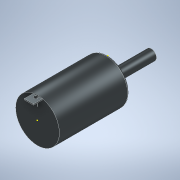
# Autodesk Inventor part: DC MOTOR
Saved by Autodesk Inventor 2022 (Build 260153000, 153)
## iProperties
Created: 2022-08-22
Part Number: DC MOTOR
Material: Iron, Gray
Document SubType Name: Modeling
Designer: Sachin
Density: 7.15 g/cm^3
Appearance: Iron Gray
Author: Sachin
Autodesk Inventor part; units mm, degrees
ref_plane "YZ Plane" through (0, 0, 0) normal (1, 0, 0) x (0, 1, 0)
ref_plane "XZ Plane" through (0, 0, 0) normal (0, 1, 0) x (-1, 0, 0)
ref_plane "XY Plane" through (0, 0, 0) normal (0, 0, 1) x (1, 0, 0)
sketch "Sketch1" plane through (0, 0, 0) normal (0, 0, 1) x (1, 0, 0)
  circle A0 centre (0, 0) radius 12.5
  dimension "d0" = 25
  constraints: 1 centre point, 1 coincident
  measures "d0" diameter of A0
extrude "Extrusion1" add sketch "Sketch1" along normal blind 40
sketch "Sketch2" plane through (0, 0, 40) normal (0, 0, 1) x (1, 0, 0)
  point P0 (0, 0)
sketch "Sketch3" plane through (0, 0, 40) normal (0, 0, 1) x (1, 0, 0)
  line L0 (-2.5708, 11.9347) -> (2.7411, 11.9347)
  line L1 (2.7411, 11.9347) -> (2.7411, 11.3559)
  line L2 (2.7411, 11.3559) -> (-2.5708, 11.3559)
  line L3 (-2.5708, 11.3559) -> (-2.5708, 11.9347)
  point P0 (0, 0)
  constraints: 8 end point, 2 parallel, 1 horizontal, 1 perpendicular
extrude "Extrusion2" add sketch "Sketch3" along normal blind 5
sketch "Sketch5" plane through (-2.5708, 11.9347, 40) normal (0, 1, 0) x (1, 0, 0)
  circle A0 centre (2.5708, -0.9862) radius 1
  point P0 (2.5708, 40)
  dimension "d9" = 2
  constraints: 1 centre point
  measures "d9" diameter of A0
extrude "Extrusion4" cut sketch "Sketch5" against normal blind 5
sketch "Sketch6" plane through (0, 0, 0) normal (0, 0, -1) x (-1, 0, 0)
  circle A0 centre (0, 0) radius 3
  constraints: 1 centre point, 1 coincident
extrude "Extrusion5" add sketch "Sketch6" along normal blind 25
fillet "Fillet1" radius 1 1 edges at (-12.5, 0, 0)
sketch "Sketch7" plane through (-2.5708, 11.9347, 45) normal (0, 1, 0) x (1, 0, 0)
  point P0 (2.5708, 45)
body "Solid1"
